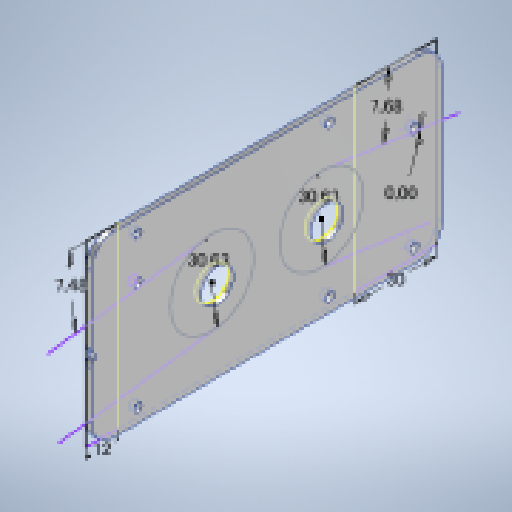
# Autodesk Inventor part: motor
Saved by Autodesk Inventor 2025 (Build 290162000, 162)
## iProperties
Created: 2025-02-25
Part Number: motor
Material: アルミニウム 6061
Document SubType Name: Modeling
Designer: Zhopa
Density: 2.7 g/cm^3
Appearance: アルミニウム - フラット
Mass: 43.0624 g
Surface Area: 169.864 cm^2
Volume: 15.949 cm^3
Author: Zhopa
Autodesk Inventor part; units mm, degrees
ref_plane "YZ Plane" through (0, 0, 0) normal (1, 0, 0) x (0, 1, 0)
ref_plane "XZ Plane" through (0, 0, 0) normal (0, 1, 0) x (-1, 0, 0)
ref_plane "XY Plane" through (0, 0, 0) normal (0, 0, 1) x (1, 0, 0)
sketch "Sketch1" plane through (0, 0, 0) normal (1, 0, 0) x (0, 1, 0)
  circle A0 centre (0, 0) radius 6
  line L0 (36, -46) -> (36, 34)
  line L1 (36, 34) -> (-29, 34)
  line L2 (-29, 34) -> (-29, -46)
  line L3 (-29, -46) -> (36, -46)
  point P0 (0, -17.5)
  point P1 (17.5, 0)
  point P2 (0, 17.5)
  point P3 (-17.5, 0)
  point P4 (0, -30)
  point P5 (0, 30)
  point P6 (31, -41)
  point P7 (31, 29)
  point P8 (-24, 29)
  point P9 (-24, -41)
  dimension "d6" = 30
  dimension "d9" = 360
  dimension "d15" = 5
  dimension "d16" = 5
  dimension "d17" = 80
  dimension "d18" = 65
  dimension "d28" = 5
  dimension "d29" = 55
  dimension "d30" = 55
  dimension "d38" = 12
  constraints: 8 end point, 3 perpendicular, 1 centre point, 1 coincident, 1 vertical, 3 other
  measures "d6" distance of point (0, -30) point (0, 0)
  measures "d15" horizontal distance of L0.start point (31, -41)
  measures "d16" horizontal distance of L0.start point (31, -41)
  measures "d17" distance of L0.start L0.end
  measures "d18" distance of L0.end L1.end
  measures "d28" distance from line of point (31, 29) L1
  measures "d29" distance of point (-24, 29) point (31, 29)
  measures "d30" distance of point (31, -41) point (-24, -41)
  measures "d38" diameter of A0
extrude "Extrusion1" add sketch "Sketch1" along normal blind 2
hole "Hole1" at (0, 31, -41) at (0, 31, 29) at (0, -24, 29) at (0, -24, -41) direction (1, 0, 0) diameter 3.2 depth 43.75 tip angle 118
sketch "Sketch2" plane through (0, 0, 0) normal (-1, 0, 0) x (0, 0, 1)
  circle A0 centre (-40, 0) radius 6
  line L0 (-46, 36) -> (34, 36) projected
  line L1 (-46, 36) -> (-52, 36)
  line L2 (-52, 36) -> (-52, -29)
  line L3 (-52, -29) -> (-46, -29)
  line L4 (-46, -29) -> (-46, 36)
  point P0 (0, 0)
  point P1 (0, 25.1294)
  point P2 (0, -32.6005)
  dimension "d31" = 40
  dimension "d32" = 12
  dimension "d33" = 6
  constraints: 8 end point, 2 parallel, 1 centre point, 1 coincident, 1 horizontal, 1 perpendicular
  measures "d31" distance of point (-40, 0) point (0, 0)
  measures "d32" diameter of A0
  measures "d33" distance of L3.end L2.end
extrude "Extrusion2" add sketch "Sketch2" against normal blind 2 contours L4 L3 L2 L1
extrude "Extrusion3" cut sketch "Sketch2" against normal blind 2 contours A0
sketch "Sketch3" plane through (0, 0, 0) normal (-1, 0, 0) x (0, 0, 1)
  line L0 (34, 36) -> (34, -29) projected
  line L1 (34, 36) -> (46, 36)
  line L2 (46, 36) -> (46, -29)
  line L3 (46, -29) -> (34, -29)
  line L4 (34, -29) -> (34, 36)
  line L5 (-52, 36) -> (-52, -29) projected
  line L6 (-52, 36) -> (-82, 36)
  line L7 (-82, 36) -> (-82, -29)
  line L8 (-82, -29) -> (-52, -29)
  line L9 (-52, -29) -> (-52, 36)
  circle A0 centre (0, 0) radius 6 projected
  circle A1 centre (0, 0) radius 15.315
  circle A2 centre (-40, 0) radius 6 projected
  circle A3 centre (-40, 0) radius 15.315
  line L10 (-40, 15.315) -> (-90.0791, 8.5618)
  line L11 (-35.9433, -14.768) -> (-79.6302, -20.6591)
  line L12 (0, 15.315) -> (59.9492, 7.4438)
  line L13 (-3.9709, -14.9288) -> (55.9782, -22.7999)
  circle A4 centre (29, 15.315) radius 1.6
  point P0 (-71.9486, -24)
  point P1 (-71.9486, 13.715)
  point P2 (-52, -29)
  dimension "d41" = 30.63
  dimension "d39" = 12
  dimension "d40" = 30
  dimension "d42" = 30.63
  dimension "d43" = 7.68
  dimension "d44" = 0
  dimension "d45" = 7.48
  constraints: 24 end point, 4 parallel, 2 centre point, 2 coincident, 2 horizontal, 2 perpendicular, 2 point on circle, 1 point on line, 1 vertical alignment, 2 other
  measures "d39" distance of L2.end L3.end
  measures "d40" distance of L8.end L7.end
  measures "d42" diameter of A3
  measures "d43" angle of L6 L10
  measures "d44" angle of L10 L11
  measures "d45" angle of L1 L12
extrude "Extrusion4" add sketch "Sketch3" against normal blind 2 contours L1 L2 L12 L0 | L12 L2 L13 L0 | L13 L2 L3 L0 | L5 L10 L7 L6 | L5 A3 L8 L7 L10 | L5 A3
hole "Hole2" at (0, -24, -71.9486) at (0, 13.715, -71.9486) at (0, 15.315, 29) direction (1, 0, 0) diameter 3.2 depth 43.75 tip angle 118
fillet "Fillet1" radius 8.25 4 edges at (1, 36, -82) (1, -29, -82) (1, -29, 46) (1, 36, 46)
sketch "Sketch4" plane through (0, 0, 0) normal (-1, 0, 0) x (0, 0, 1)
  line L0 (46, -20.75) -> (46, 27.75) projected
  point P0 (0, 0)
  point P1 (46, 0)
  constraints: 1 point on line
hole "Hole3" at (0, 0, 46) direction (1, 0, 0) diameter 3.2 depth 43.75 tip angle 118
fillet "Fillet2" radius 2 2 edges at (1, 1.6, 46) (1, -1.6, 46)
body "Solid1"
